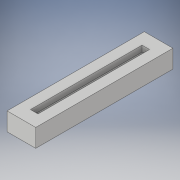
# Autodesk Inventor part: Linear Resistor Body
Saved by Autodesk Inventor 2019 (Build 230136000, 136)
## iProperties
Created: 2019-02-19
Part Number: Linear Resistor Body
Material: Generic
Document SubType Name: Modeling
Designer: Jared
Density: 1 g/cm^3
Appearance: Default
Author: Jared
Autodesk Inventor part; units mm, degrees
ref_plane "YZ Plane" through (0, 0, 0) normal (1, 0, 0) x (0, 1, 0)
ref_plane "XZ Plane" through (0, 0, 0) normal (0, 1, 0) x (-1, 0, 0)
ref_plane "XY Plane" through (0, 0, 0) normal (0, 0, 1) x (1, 0, 0)
sketch "Sketch1" plane through (0, 0, 0) normal (0, 1, 0) x (-1, 0, 0)
  line L0 (0, 0) -> (9.5, 0)
  line L1 (9.5, 0) -> (9.5, -45.5)
  line L2 (9.5, -45.5) -> (0, -45.5)
  line L3 (0, -45.5) -> (0, 0)
  dimension "d0" = 9.5
  dimension "d1" = 45.5
  constraints: 8 end point, 2 parallel, 1 horizontal, 1 perpendicular
  measures "d0" distance of L1.end L2.end
  measures "d1" distance of L0.end L1.end
extrude "Extrusion1" add sketch "Sketch1" along normal blind 6
sketch "Sketch2" plane through (0, 6, 0) normal (0, 1, 0) x (1, 0, 0)
  line L0 (-9.5, 0) -> (0, 0) projected
  line L1 (0, 0) -> (0, 45.5) projected
  line L2 (0, 45.5) -> (-9.5, 45.5) projected
  line L3 (-9.5, 45.5) -> (-9.5, 0) projected
  line L4 (-6, 4.25) -> (-3.5, 4.25)
  line L5 (-3.5, 4.25) -> (-3.5, 41.25)
  line L6 (-3.5, 41.25) -> (-6, 41.25)
  line L7 (-6, 41.25) -> (-6, 4.25)
  line L8 (-4.75, 41.25) -> (-4.75, 45.5)
  line L9 (0, 45.5) -> (-9.5, 45.5) projected
  line L10 (-6, 22.75) -> (-9.5, 22.75)
  line L11 (-9.5, 45.5) -> (-9.5, 0) projected
  line L12 (-4.75, 4.25) -> (-4.75, 0)
  line L13 (-9.5, 0) -> (0, 0) projected
  line L14 (-3.5, 22.75) -> (0, 22.75)
  dimension "d4" = 2.5
  dimension "d5" = 37
  constraints: 16 end point, 8 midpoint, 3 perpendicular, 2 collinear, 2 parallel, 2 point on line, 1 horizontal
  measures "d4" distance of L6.end L5.end
  measures "d5" distance of L5.end L4.end
extrude "Extrusion2" cut sketch "Sketch2" against normal blind 2 contours L4 L7 L6 L5
body "Solid1"
